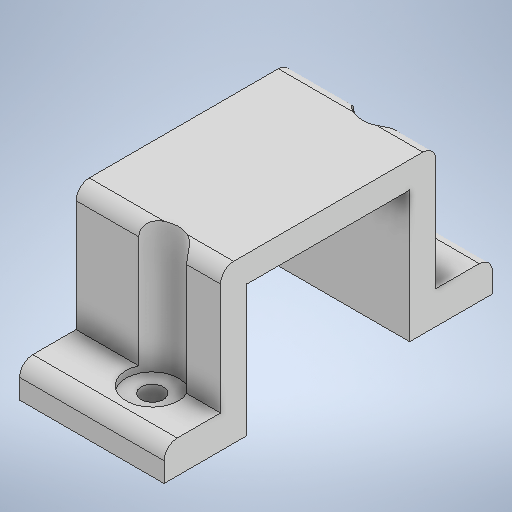
# Autodesk Inventor part: soporte velo
Saved by Autodesk Inventor 2025 (Build 290162000, 162)
## iProperties
Created: 2024-10-10
Part Number: soporte velo
Material: Generic
Document SubType Name: Modeling
Designer: Zoe
Density: 1 g/cm^3
Appearance: Default
Author: Zoe
Autodesk Inventor part; units mm, degrees
ref_plane "YZ Plane" through (0, 0, 0) normal (1, 0, 0) x (0, 1, 0)
ref_plane "XZ Plane" through (0, 0, 0) normal (0, 1, 0) x (-1, 0, 0)
ref_plane "XY Plane" through (0, 0, 0) normal (0, 0, 1) x (1, 0, 0)
sketch "Sketch1" plane through (0, 0, 0) normal (1, 0, 0) x (0, 1, 0)
  line L0 (-2.5, 12.5) -> (-5, 12.5)
  line L1 (5, -6.2) -> (5, 6.2)
  line L2 (-5, 12.5) -> (-5, 6.2)
  line L3 (-5, -6.2) -> (-5, -12.5)
  line L4 (-5, 6.2) -> (5, 6.2)
  line L5 (-5, -6.2) -> (5, -6.2)
  line L6 (7, -6.2) -> (7, 8.2)
  line L7 (5, 6.2) -> (5, -6.2)
  line L8 (5, 6.2) -> (-5, 6.2)
  line L9 (-5, 6.2) -> (-5, 8.2)
  line L10 (-2.5, 8.2) -> (7, 8.2)
  line L11 (7, 8.2) -> (7, 6.2)
  line L12 (-5, 6.2) -> (-2.5, 6.2)
  line L13 (-2.5, 8.2) -> (-2.5, 12.5)
  line L14 (-2.5, 12.5) -> (-5, 12.5)
  line L15 (-5, 12.5) -> (-5, 6.2)
  line L16 (5, 6.2) -> (5, 0)
  line L17 (5, 0) -> (-5.8889, 0)
  line L18 (-2.5, -12.5) -> (-5, -12.5)
  line L19 (5, 6.2) -> (5, -6.2)
  line L20 (-5, -12.5) -> (-5, -6.2)
  line L21 (-5, -6.2) -> (5, -6.2)
  line L22 (7, 6.2) -> (7, -8.2)
  line L23 (5, -6.2) -> (5, 6.2)
  line L24 (5, -6.2) -> (-5, -6.2)
  line L25 (-5, -6.2) -> (-5, -8.2)
  line L26 (-2.5, -8.2) -> (7, -8.2)
  line L27 (7, -8.2) -> (7, -6.2)
  line L28 (-5, -6.2) -> (-2.5, -6.2)
  line L29 (-2.5, -8.2) -> (-2.5, -12.5)
  line L30 (-2.5, -12.5) -> (-5, -12.5)
  line L31 (-5, -12.5) -> (-5, -6.2)
  line L32 (5, -6.2) -> (5, 0)
  dimension "d1" = 25
  dimension "d2" = 6.3
  dimension "d5" = 10
  dimension "d6" = 10
  dimension "d9" = 2
  dimension "d10" = 2.5
  dimension "d11" = 6.2
  constraints: 66 end point, 13 symmetric about line, 5 parallel, 4 point on line, 3 horizontal, 3 perpendicular, 2 midpoint, 1 collinear
  measures "d1" distance of L3.end L0.end
  measures "d2" distance of L0.end L2.end
  measures "d5" distance of L1.end L2.end
  measures "d6" distance of L1.start L3.start
  measures "d9" distance of L8.end L9.end
  measures "d10" distance of L0.start L14.end
  measures "d11" distance of L1.end L16.end
extrude "Extrusion1" add sketch "Sketch1" along normal blind 11
sketch "Sketch2" plane through (0, -2.5, 12.5) normal (0, 1, 0) x (1, 0, 0)
  line L0 (0, 4.3) -> (0, 0) projected
  line L1 (0, 0) -> (11, 0) projected
  line L2 (6.6, 0) -> (6.6, 3.5)
  line L3 (6.6, 3.5) -> (0, 3.5)
  point P0 (0, 12.5)
  dimension "d15" = 3.5
  dimension "d16" = 6.6
  constraints: 4 end point, 2 perpendicular, 2 point on line, 1 coincident
  measures "d15" distance of L2.start L2.end
  measures "d16" distance of L2.end L3.end
hole "Hole1" at (6.6, -2.5, 9) direction (0, -1, 0) diameter 1.7 depth 5.692
sketch "Sketch3" plane through (0, -2.5, -8.2) normal (0, 1, 0) x (1, 0, 0)
  line L0 (0, 4.3) -> (11, 4.3) projected
  line L1 (0, 4.3) -> (6.6, 4.3)
  line L2 (6.6, 4.3) -> (6.6, 0.8)
  line L3 (6.6, 4.3) -> (10.1, 4.3) construction
  point P0 (0, -8.2)
  dimension "d24" = 6.6
  dimension "d25" = 3.5
  dimension "d26" = 90
  constraints: 6 end point, 1 coincident, 1 horizontal, 1 perpendicular, 1 point on line, 1 vertical
  measures "d24" distance of L0.start L1.end
  measures "d25" distance of L1.end L2.end
  measures "d26" angle of L2 L3
hole "Hole2" at (6.6, -2.5, -9) direction (0, -1, 0) diameter 1.7 depth 5.692
sketch "Sketch4" plane through (0, 7, 8.2) normal (0, 1, 0) x (1, 0, 0)
  arc A0 (6.3128, 0) -> (6.8872, 0) centre (6.6, -0.8) ccw projected
  arc A1 (6.8872, 16.4) -> (6.3128, 16.4) centre (6.6, 17.2) ccw projected
  point P0 (0, 8.2)
  constraints: 2 coincident
hole "Hole3" at (6.6, 7, 9) at (6.6, 7, -9) direction (0, -1, 0) diameter 4 depth 10
fillet "Fillet1" radius 1 6 edges at (2.3835, 7, -8.2) (2.3835, 7, 8.2) (9.7165, 7, 8.2) (9.7165, 7, -8.2) (5.5, -2.5, 12.5) (5.5, -2.5, -12.5)
sketch "Sketch5" plane through (0, 5, -6.2) normal (0, -1, 0) x (1, 0, 0)
  line L0 (11, 12.4) -> (11, 0) projected
  line L1 (0, 12.4) -> (11, 12.4) projected
  line L2 (11, 12.4) -> (10, 12.4)
  line L3 (10, 12.4) -> (6, 12.4)
  line L4 (0, 0) -> (11, 0) projected
  line L5 (10, 12.4) -> (6, 12.4)
  line L6 (6, 12.4) -> (6, 0)
  line L7 (6, 0) -> (10, 0)
  line L8 (10, 0) -> (10, 12.4)
  point P0 (0, 6.2)
  point P1 (10, 0)
  dimension "d42" = 1
  dimension "d43" = 4
  constraints: 12 end point, 3 point on line, 2 parallel, 1 horizontal, 1 perpendicular
  measures "d42" distance of L0.start L2.end
  measures "d43" distance of L2.end L3.end
extrude "Extrusion2" add sketch "Sketch5" along normal blind 0.5 contours L8 L4 L6 L1
fillet "Fillet2" radius 0.3 2 edges at (10, 4.5, 0) (6, 4.5, 0)
body "Solid1"
